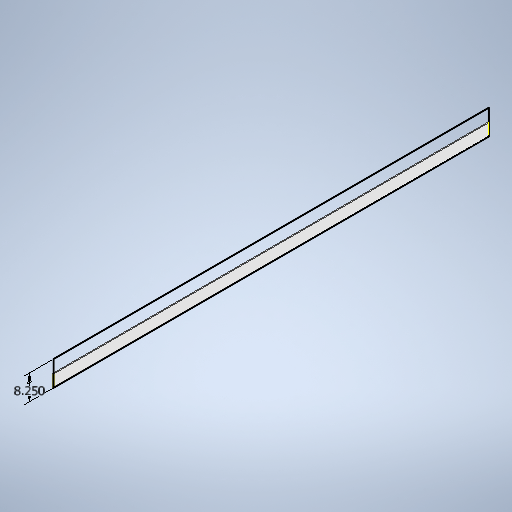
# Autodesk Inventor part: Fiber_Cement_Board_With_Height_3_Inches
Saved by Autodesk Inventor 2025 (Build 290162010, 162A)
## iProperties
Created: 2024-09-16
Part Number: Fiber_Cement_Board_With_Height_3_Inches
Material: Generic
Document SubType Name: Modeling
Designer: Tom
Density: 1 g/cm^3
Appearance: White
Author: Tom
Autodesk Inventor part; units mm, degrees
ref_plane "YZ Plane" through (0, 0, 0) normal (1, 0, 0) x (0, 1, 0)
ref_plane "XZ Plane" through (0, 0, 0) normal (0, 1, 0) x (-1, 0, 0)
ref_plane "XY Plane" through (0, 0, 0) normal (0, 0, 1) x (1, 0, 0)
sketch "Sketch1" plane through (0, 0, 0) normal (1, 0, 0) x (0, 1, 0)
  line L0 (0, 0) -> (100.4316, 0)
  line L1 (100.4316, 0) -> (100.4316, 3657.6)
  line L2 (100.4316, 3657.6) -> (0, 3657.6)
  line L3 (0, 3657.6) -> (0, 0)
  dimension "d0" = 3657.6
  dimension "d1" = 100.4316
  constraints: 8 end point, 2 parallel, 1 horizontal, 1 perpendicular
  measures "d0" distance of L2.end L0.start
  measures "d1" distance of L0.start L0.end
extrude "Extrusion1" add sketch "Sketch1" along normal blind 7.9375
sketch "Sketch2" plane through (7.9375, 0, 0) normal (1, 0, 0) x (0, 0, -1)
  line L0 (-3657.6, 100.4316) -> (-3657.6, 0) projected
  line L1 (-3657.6, 0) -> (0, 0)
  line L2 (0, 0) -> (0, 209.55)
  line L3 (0, 209.55) -> (-3657.6, 209.55)
  line L4 (-3657.6, 209.55) -> (-3657.6, 0)
  line L5 (0, 0) -> (0, 100.4316) projected
  dimension "d4" = 209.55
  constraints: 8 end point, 2 parallel, 1 collinear, 1 horizontal, 1 perpendicular
  measures "d4" distance of L3.end L0.end
body "Solid1"
